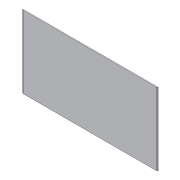
# Autodesk Inventor part: GE-12018
Saved by Autodesk Inventor 2012 (Build 160160000, 160)
## iProperties
Created: 2011-06-06
Part Number: GE-12018
Document SubType Name: Modeling
Designer: dfoster
Density: 1 g/cm^3
Mass: 33708.8 g
Surface Area: 54103.9 cm^2
Volume: 33708.8 cm^3
Description: Bridge Deck
Material: Default
Title: Bridge Deck
Author: dfoster
Autodesk Inventor part; units mm, degrees
ref_plane "YZ Plane" through (0, 0, 0) normal (1, 0, 0) x (0, 1, 0)
ref_plane "XZ Plane" through (0, 0, 0) normal (0, 1, 0) x (-1, 0, 0)
ref_plane "XY Plane" through (0, 0, 0) normal (0, 0, 1) x (1, 0, 0)
sketch "Sketch1" plane through (0, 0, 0) normal (0, 0, 1) x (1, 0, 0)
  line L0 (0, 0) -> (2235.2, 0)
  line L1 (2235.2, 0) -> (2235.2, 1193.8)
  line L2 (2235.2, 1193.8) -> (0, 1193.8)
  line L3 (0, 1193.8) -> (0, 0)
  dimension "d0" = 1193.8
  dimension "d1" = 2235.2
  constraints: 8 end point, 2 parallel, 1 horizontal, 1 perpendicular
  measures "d0" distance between parallel lines of L0 L2
  measures "d1" distance between parallel lines of L1 L3
extrude "Extrusion1" add sketch "Sketch1" along normal blind 12.7
chamfer "Chamfer1" distance 6.35 angle 75 1 edges at (2235.2, 596.9, 12.7) measured on face at (2235.2, 397.9333, 4.2333)
chamfer "Chamfer3" distance 6.35 angle 75 1 edges at (0, 596.9, 12.7) measured on face at (0, 795.8667, 4.2333)
body "Solid1"
